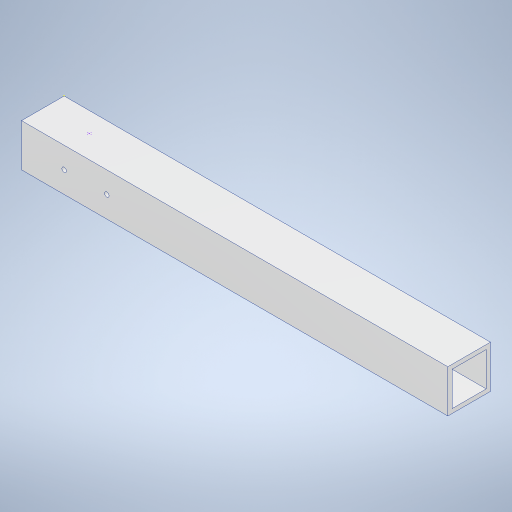
# Autodesk Inventor part: base
Saved by Autodesk Inventor 2024 (Build 280153000, 153)
## iProperties
Created: 2025-06-07
Part Number: base
Material: アルミニウム 6061
Document SubType Name: Modeling
Designer: HosodaLab2
Density: 2.7 g/cm^3
Appearance: アルミニウム - フラット
Author: HosodaLab2
Autodesk Inventor part; units mm, degrees
ref_plane "YZ Plane" through (0, 0, 0) normal (1, 0, 0) x (0, 1, 0)
ref_plane "XZ Plane" through (0, 0, 0) normal (0, 1, 0) x (-1, 0, 0)
ref_plane "XY Plane" through (0, 0, 0) normal (0, 0, 1) x (1, 0, 0)
sketch "スケッチ1" plane through (0, 0, 0) normal (0, 1, 0) x (-1, 0, 0)
  line L0 (0, 0) -> (-30, 0)
  line L1 (-30, 0) -> (-30, -30)
  line L2 (-30, -30) -> (0, -30)
  line L3 (0, -30) -> (0, 0)
  line L4 (-3, -3) -> (-27, -3)
  line L5 (-27, -3) -> (-27, -27)
  line L6 (-27, -27) -> (-3, -27)
  line L7 (-3, -27) -> (-3, -3)
  dimension "d0" = 30
  dimension "d1" = 30
  dimension "d2" = 24
  dimension "d3" = 24
  dimension "d4" = 3
  dimension "d5" = 3
  constraints: 16 end point, 4 parallel, 2 horizontal, 2 perpendicular
  measures "d0" distance of L2.end L1.end
  measures "d1" distance of L0.end L1.end
  measures "d2" distance of L6.end L5.end
  measures "d3" distance of L5.end L4.end
  measures "d4" distance between parallel lines of L2 L6
  measures "d5" distance between parallel lines of L3 L7
extrude "押し出し1" add sketch "スケッチ1" along normal blind 300
sketch "スケッチ2" plane through (0, 0, 0) normal (0, 0, 1) x (1, 0, 0)
  point P0 (0, 0)
  point P1 (13.8561, 31.5859)
sketch "スケッチ3" plane through (30, 0, 0) normal (1, 0, 0) x (0, 0, -1)
  line L0 (30, 0) -> (30, 300) projected
  line L1 (0, 0) -> (30, 0) projected
  point P0 (15, 60)
  point P1 (15, 30)
  point P2 (15, 0)
  dimension "d11" = 30
  dimension "d12" = 30
  constraints: 1 midpoint
  measures "d11" distance of point (15, 30) point (15, 60)
  measures "d12" distance of point (15, 0) point (15, 30)
hole "穴1" at (30, 30, -15) at (30, 60, -15) direction (-1, 0, 0) diameter 3.2 end through all
